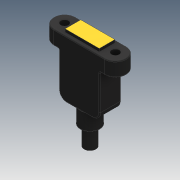
# Autodesk Inventor part: hdmi-cable
Saved by Autodesk Inventor 2017 (Build 210142000, 142)
## iProperties
Created: 2018-08-17
Part Number: hdmi-cable
Material: Rubber
Document SubType Name: Modeling
Designer: Luiz Gustavo
Density: 0.93 g/cm^3
Appearance: Rubber - Black
Author: Luiz Gustavo
Autodesk Inventor part; units mm, degrees
ref_plane "YZ Plane" through (0, 0, 0) normal (1, 0, 0) x (0, 1, 0)
ref_plane "XZ Plane" through (0, 0, 0) normal (0, 1, 0) x (-1, 0, 0)
ref_plane "XY Plane" through (0, 0, 0) normal (0, 0, 1) x (1, 0, 0)
sketch "Sketch1" plane through (0, 0, 0) normal (0, 0, 1) x (1, 0, 0)
  line L0 (-13, 0) -> (13, 0) construction
  line L1 (-13, -5.5) -> (13, -5.5)
  line L2 (13, 5.5) -> (-13, 5.5)
  arc A0 (-13, 5.5) -> (-13, -5.5) centre (-13, 0) ccw
  arc A1 (13, -5.5) -> (13, 5.5) centre (13, 0) ccw
  circle A2 centre (-13, 0) radius 2
  circle A3 centre (13, 0) radius 2
  line L3 (-8.75, 4) -> (8.75, 4)
  line L4 (8.75, 4) -> (8.75, -4)
  line L5 (8.75, -4) -> (-8.75, -4)
  line L6 (-8.75, -4) -> (-8.75, 4)
  line L7 (-8.75, 4) -> (8.75, -4) construction
  line L8 (8.75, 4) -> (-8.75, -4) construction
  line L9 (-10.5, 5.5) -> (10.5, 5.5)
  line L10 (10.5, 5.5) -> (10.5, -5.5)
  line L11 (10.5, -5.5) -> (-10.5, -5.5)
  line L12 (-10.5, -5.5) -> (-10.5, 5.5)
  line L13 (-10.5, 5.5) -> (10.5, -5.5) construction
  line L14 (10.5, 5.5) -> (-10.5, -5.5) construction
  circle A4 centre (0, 0) radius 5
  circle A5 centre (0, 0) radius 3
  dimension "d0" = 11
  dimension "d1" = 37
  dimension "d2" = 4
  dimension "d3" = 17.5
  dimension "d4" = 8
  dimension "d5" = 21
  dimension "d6" = 11
  dimension "d7" = 10
  dimension "d8" = 6
  constraints: 32 end point, 6 centre point, 5 midpoint, 5 parallel, 4 coincident, 4 point on circle, 4 tangent, 3 horizontal, 2 perpendicular, 1 equal radius
  measures "d0" distance between parallel lines of L2 L1
  measures "d2" diameter of A2
  measures "d3" distance of L4.end L5.end
  measures "d4" distance of L3.end L4.end
  measures "d5" distance of L10.end L11.end
  measures "d6" distance of L9.end L10.end
  measures "d7" diameter of A4
  measures "d8" diameter of A5
extrude "Extrusion1" add sketch "Sketch1" along normal blind 7.5 contours A0 L2 L12 L1 | L12 L2 L10 L1 | L10 L2 A1 L1 | L3 A4 L5 L6 | A4 L3 | L3 A4 L5 | L3 L4 L5 A4 | L5 A4 | A5
extrude "Extrusion2" add sketch "Sketch1" along normal blind 9 contours L3 A4 L5 L6 | L3 A4 L5 | L3 L4 L5 A4 | A5
extrude "Extrusion3" add sketch "Sketch1" against normal blind 22 contours L12 L2 L10 L1 | L3 A4 L5 L6 | A4 L3 | L3 A4 L5 | L3 L4 L5 A4 | L5 A4 | A5
extrude "Extrusion4" add sketch "Sketch1" against normal blind 31 contours A4 L3 | L3 A4 L5 | L5 A4 | A5
extrude "Extrusion5" add sketch "Sketch1" against normal blind 40.5 contours A5
fillet "Fillet1" radius 4 2 edges at (10.5, 0, -22) (-10.5, 0, -22)
fillet "Fillet2" radius 0.5 25 edges at (10.5, 0, 0) (-10.5, 0, 0) (-5, 0, -22) (-5, 0, -31) (-3, 0, -31) (11.75, 5.5, 0) (11.75, -5.5, 0) (18.5, 0, 0) (-11.75, -5.5, 0) (-11.75, 5.5, 0) (-18.5, 0, 0) (-9.3284, 5.5, -20.8284) (0, 5.5, -22) (9.3284, 5.5, -20.8284) (10.5, 5.5, -9) (-10.5, 5.5, -9) (9.3284, -5.5, -20.8284) (0, -5.5, -22) (-9.3284, -5.5, -20.8284) (-10.5, -5.5, -9) (10.5, -5.5, -9) (0, 5.5, 7.5) (-18.5, 0, 7.5) (0, -5.5, 7.5) (18.5, 0, 7.5)
body "Solid1"
